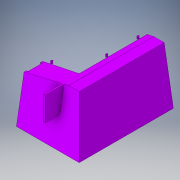
# Autodesk Inventor part: CPURightOne
Saved by Autodesk Inventor 2019 (Build 230136000, 136)
## iProperties
Created: 2019-01-04
Part Number: CPURightOne
Material: Generic
Document SubType Name: Modeling
Designer: james
Density: 1 g/cm^3
Appearance: Default(1)
Author: james
Autodesk Inventor part; units mm, degrees
ref_plane "YZ Plane" through (0, 0, 0) normal (1, 0, 0) x (0, 1, 0)
ref_plane "XZ Plane" through (0, 0, 0) normal (0, 1, 0) x (-1, 0, 0)
ref_plane "XY Plane" through (0, 0, 0) normal (0, 0, 1) x (1, 0, 0)
sketch "Sketch1" plane through (0, 0, 0) normal (0, 1, 0) x (-1, 0, 0)
  line L0 (8.325, 64.7833) -> (-61.525, 64.7833)
  line L1 (-61.525, 64.7833) -> (-61.525, -81.2667)
  line L2 (-61.525, -81.2667) -> (8.325, -81.2667)
  line L3 (8.325, -81.2667) -> (8.325, 64.7833)
  point P0 (0, 0)
  dimension "d0" = 146.05
  dimension "d1" = 69.85
  constraints: 8 end point, 2 parallel, 1 horizontal, 1 perpendicular
  measures "d0" distance of L0.end L1.end
  measures "d1" distance of L1.end L2.end
extrude "Extrusion1" add sketch "Sketch1" along normal blind 5.08
sketch "Sketch2" plane through (61.525, 0, 64.7833) normal (1, 0, 0) x (0, 0, -1)
  line L0 (0, 5.08) -> (146.05, 5.08) projected
  line L1 (0, 5.08) -> (5.08, 5.08)
  line L2 (5.08, 5.08) -> (5.08, 71.12)
  line L3 (5.08, 71.12) -> (0, 71.12)
  line L4 (0, 71.12) -> (0, 5.08)
  line L5 (0, 0) -> (146.05, 0) projected
  point P0 (64.7833, 0)
  dimension "d4" = 5.08
  dimension "d5" = 71.12
  constraints: 8 end point, 2 parallel, 1 horizontal, 1 perpendicular
  measures "d4" distance between parallel lines of L4 L2
  measures "d5" distance between parallel lines of L5 L3
extrude "Extrusion2" add sketch "Sketch2" against normal blind 69.85
sketch "Sketch3" plane through (61.525, 0, -81.2667) normal (0, 0, -1) x (-1, 0, 0)
  line L0 (0, 5.08) -> (69.85, 5.08) projected
  line L1 (0, 0) -> (69.85, 0) projected
  line L2 (0, 5.08) -> (5.08, 5.08)
  line L3 (5.08, 5.08) -> (5.08, 71.12)
  line L4 (5.08, 71.12) -> (0, 71.12)
  line L5 (0, 71.12) -> (0, 5.08)
  point P0 (61.525, 0)
  dimension "d8" = 5.08
  dimension "d9" = 71.12
  constraints: 8 end point, 2 parallel, 1 horizontal, 1 perpendicular
  measures "d8" distance between parallel lines of L5 L3
  measures "d9" distance between parallel lines of L1 L4
extrude "Extrusion3" add sketch "Sketch3" against normal blind 146.05
sketch "Sketch4" plane through (61.525, 71.12, 64.7833) normal (0, 1, 0) x (1, 0, 0)
  line L0 (-5.08, 5.08) -> (-69.85, 5.08) projected
  line L1 (-5.08, 146.05) -> (-5.08, 5.08) projected
  line L2 (-69.85, 5.08) -> (-5.08, 5.08) projected
  line L3 (-69.85, 5.08) -> (-69.85, -19.05)
  line L4 (-69.85, -19.05) -> (19.05, -19.05)
  line L5 (19.05, -19.05) -> (19.05, 146.05)
  line L6 (19.05, 146.05) -> (-5.08, 146.05)
  line L7 (-5.08, 5.08) -> (-5.08, 146.05) projected
  line L8 (-5.08, 5.08) -> (-5.08, 146.05)
  line L9 (-5.08, 5.08) -> (-69.85, 5.08)
  point P0 (-61.525, 64.7833)
  dimension "d12" = 24.13
  dimension "d13" = 24.13
  constraints: 12 end point, 3 perpendicular, 2 collinear, 1 vertical
  measures "d12" distance between parallel lines of L0 L4
  measures "d13" distance of L5.end L1.start
extrude "Extrusion4" add sketch "Sketch4" against normal blind 5.08
sketch "Sketch5" plane through (-8.325, 71.12, 59.7033) normal (0, 1, 0) x (1, 0, 0)
  line L0 (88.9, -24.13) -> (88.9, 140.97) projected
  line L1 (0, -24.13) -> (88.9, -24.13) projected
  point P0 (8.325, 59.7033)
  point P1 (12.7, -14.605)
  point P2 (79.375, 52.07)
  point P3 (79.375, 128.27)
  dimension "d16" = 9.525
  dimension "d17" = 9.525
  dimension "d18" = 76.2
  dimension "d19" = 76.2
  dimension "d20" = 9.525
  dimension "d21" = 76.2
  measures "d16" distance from line of L0 point (79.375, 52.07)
  measures "d17" distance from line of L1 point (12.7, -14.605)
  measures "d18" distance from line of point (12.7, -14.605) L0
  measures "d19" distance from line of L1 point (79.375, 52.07)
  measures "d20" distance from line of L0 point (79.375, 128.27)
  measures "d21" distance of point (79.375, 52.07) point (79.375, 128.27)
hole "Hole1" at (4.375, 71.12, 74.3083) at (71.05, 71.12, 7.6333) at (71.05, 71.12, -68.5667) direction (0, -1, 0) diameter 4.826 end through all
sketch "Sketch6" plane through (-8.325, 0, -81.2667) normal (-1, 0, 0) x (0, 0, 1)
  line L0 (223.52, 0) -> (228.6, 0)
  line L1 (0, 0) -> (0, 5.08) projected
  line L2 (146.05, 0) -> (146.05, 66.04) projected
  line L3 (223.52, 0) -> (201.1265, 127)
  line L4 (201.1265, 127) -> (206.2065, 127)
  line L5 (206.2065, 127) -> (228.6, 0)
  point P0 (81.2667, 0)
  dimension "d29" = 228.6
  dimension "d30" = 5.08
  dimension "d32" = 10
  dimension "d33" = 5.08
  dimension "d34" = 127
  constraints: 8 end point, 2 horizontal
  measures "d29" distance from line of L1 L0.end
  measures "d30" distance of L0.start L0.end
  measures "d32" angle of L2 L3
  measures "d33" distance of L3.end L4.end
  measures "d34" distance between parallel lines of L0 L4
extrude "Extrusion5" add sketch "Sketch6" against normal blind 152.4
sketch "Sketch7" plane through (61.525, 0, -81.2667) normal (0, 0, -1) x (-1, 0, 0)
  line L0 (-82.55, 0) -> (-77.47, 0)
  line L1 (69.85, 0) -> (-82.55, 0) projected
  line L2 (-77.47, 0) -> (-55.0765, 127)
  line L3 (0, 0) -> (0, 66.04) projected
  line L4 (69.85, 127) -> (-82.55, 127) projected
  line L5 (-55.0765, 127) -> (-60.1565, 127)
  line L6 (-60.1565, 127) -> (-82.55, 0)
  point P0 (61.525, 0)
  dimension "d37" = 5.08
  dimension "d38" = 10
  dimension "d39" = 5.08
  constraints: 8 end point, 3 point on line
  measures "d37" distance of L0.start L0.end
  measures "d38" angle of L2 L3
  measures "d39" distance of L5.end L2.end
extrude "Extrusion6" add sketch "Sketch7" against normal blind 228.6
sketch "Sketch8" plane through (61.525, 0, -81.2667) normal (0, 0, -1) x (-1, 0, 0)
  line L0 (-60.1565, 127) -> (-82.55, 0) projected
  line L1 (-60.1565, 127) -> (-82.55, 127) projected
  line L2 (-82.55, 0) -> (-82.55, 127) projected
  point P0 (61.525, 0)
extrude "Extrusion7" cut sketch "Sketch8" against normal blind 228.6
sketch "Sketch9" plane through (-8.325, 0, -81.2667) normal (-1, 0, 0) x (0, 0, 1)
  line L0 (228.6, 0) -> (206.2065, 127) projected
  line L1 (206.2065, 127) -> (228.6, 127) projected
  line L2 (228.6, 127) -> (228.6, 0) projected
  point P0 (81.2667, 0)
extrude "Extrusion8" cut sketch "Sketch9" against normal blind 228.6
sketch "Sketch10" plane through (61.525, 0, -81.2667) normal (0, 0, -1) x (-1, 0, 0)
  line L0 (-60.1565, 127) -> (-82.55, 0) projected
  line L1 (-60.1565, 127) -> (-34.7565, 127)
  line L2 (-34.7565, 127) -> (-34.7565, 121.92)
  line L3 (-34.7565, 121.92) -> (-60.1565, 121.92)
  line L4 (-60.1565, 121.92) -> (-60.1565, 127)
  point P0 (61.525, 0)
  dimension "d46" = 25.4
  dimension "d47" = 5.08
  constraints: 8 end point, 2 parallel, 1 horizontal, 1 perpendicular
  measures "d46" distance of L2.end L3.end
  measures "d47" distance between parallel lines of L3 L1
extrude "Extrusion9" add sketch "Sketch10" against normal blind 204.7875
sketch "Sketch13" plane through (61.525, 0, -81.2667) normal (0, 0, -1) x (-1, 0, 0)
  line L0 (-34.7565, 127) -> (-60.1565, 127) projected
  line L1 (-34.7565, 127) -> (65.3895, 106.1149)
  line L2 (65.3895, 106.1149) -> (65.3895, 101.0349)
  line L3 (-34.7565, 127) -> (-34.7565, 121.92) projected
  line L4 (-34.7565, 127) -> (-34.7565, 121.92)
  line L5 (-34.7565, 121.92) -> (65.3895, 101.0349)
  point P0 (61.525, 0)
  dimension "d50" = 5.08
  dimension "d51" = 168.22
  constraints: 8 end point, 1 collinear, 1 perpendicular
  measures "d50" distance of L1.end L2.end
  measures "d51" angle of L0 L1
extrude "Extrusion10" add sketch "Sketch13" against normal blind 204.7875
sketch "Sketch14" plane through (-8.325, 0, -81.2667) normal (-1, 0, 0) x (0, 0, 1)
  line L0 (0, 66.04) -> (165.1, 66.04) projected
  line L1 (165.1, 66.04) -> (170.18, 66.04)
  line L2 (170.18, 66.04) -> (170.18, 144.8486)
  line L3 (165.1, 66.04) -> (165.1, 144.8486)
  line L4 (165.1, 144.8486) -> (170.18, 144.8486)
  point P0 (81.2667, 0)
  dimension "d54" = 5.08
  constraints: 8 end point, 2 perpendicular, 1 horizontal, 1 vertical
  measures "d54" distance between parallel lines of L2 L3
extrude "Extrusion11" add sketch "Sketch14" against normal blind 201.6125
sketch "Sketch15" plane through (61.525, 0, -81.2667) normal (0, 0, -1) x (-1, 0, 0)
  line L0 (-19.05, 66.04) -> (-65.8254, 66.04) projected
  line L1 (-19.05, 66.04) -> (-24.13, 66.04)
  line L2 (-24.13, 66.04) -> (-24.13, 144.9245)
  line L3 (-24.13, 144.9245) -> (-19.05, 144.9245)
  line L4 (-19.05, 144.9245) -> (-19.05, 66.04)
  point P0 (61.525, 0)
  dimension "d57" = 5.08
  constraints: 8 end point, 2 parallel, 1 horizontal, 1 perpendicular
  measures "d57" distance between parallel lines of L2 L4
extrude "Extrusion12" add sketch "Sketch15" against normal blind 252.4125
sketch "Sketch18" plane through (-8.325, 71.12, 83.8333) normal (0, 0, -1) x (-1, 0, 0)
  line L0 (-4.4605, 34.9949) -> (-88.9, 52.6045) projected
  line L1 (-88.9, 52.6045) -> (26.3817, 28.5629)
  line L2 (-88.9, 52.6045) -> (-88.9, 80.9754)
  line L3 (-88.9, 80.9754) -> (26.3817, 80.9754)
  line L4 (26.3817, 80.9754) -> (26.3817, 28.5629)
  point P0 (-8.325, -71.12)
  constraints: 8 end point, 2 perpendicular, 1 collinear, 1 vertical
extrude "Extrusion14" cut sketch "Sketch18" against normal blind 133.35
sketch "Sketch19" plane through (61.525, 0, -81.2667) normal (0, 0, -1) x (-1, 0, 0)
  line L0 (-19.05, 66.04) -> (-19.05, 123.7245) projected
  line L1 (-24.13, 124.7839) -> (-34.7565, 127) projected
  line L2 (-19.05, 123.7245) -> (-34.7565, 127)
  line L3 (-34.7565, 127) -> (-82.8145, 127)
  line L4 (-82.8145, 127) -> (-82.8145, 152.1406)
  line L5 (-82.8145, 152.1406) -> (-18.2912, 151.7847)
  line L6 (-18.2912, 151.7847) -> (-19.05, 123.7245)
  point P0 (61.525, 0)
  constraints: 10 end point, 1 collinear, 1 horizontal, 1 perpendicular
extrude "Extrusion15" cut sketch "Sketch19" against normal blind 338.1375
sketch "Sketch21" plane through (0, 5.08, 0) normal (0, 1, 0) x (1, 0, 0)
  line L0 (56.445, -59.7033) -> (56.445, 81.2667) projected
  line L1 (56.445, 81.2667) -> (-8.325, 81.2667) projected
  line L2 (-8.325, 81.2667) -> (-8.325, -59.7033) projected
  line L3 (-8.325, -59.7033) -> (56.445, -59.7033) projected
  point P0 (0, 0)
extrude "Extrusion16" cut sketch "Sketch21" along normal blind 338.1375
sketch "Sketch22" plane through (-8.325, 71.12, 59.7033) normal (0, 1, 0) x (1, 0, 0)
  circle A0 centre (79.375, 52.07) radius 2.413 projected
  circle A1 centre (12.7, -14.605) radius 2.413 projected
  circle A2 centre (79.375, 128.27) radius 2.413 projected
  line L0 (64.77, 0) -> (0, 0) projected
  line L1 (0, 0) -> (0, -24.13) projected
  line L2 (0, -24.13) -> (88.9, -24.13) projected
  line L3 (88.9, -24.13) -> (88.9, 140.97) projected
  line L4 (64.77, 140.97) -> (88.9, 140.97) projected
  line L5 (64.77, 140.97) -> (64.77, 0) projected
  point P0 (8.325, 59.7033)
extrude "Extrusion17" cut sketch "Sketch22" along normal blind 338.1375
sketch "Sketch23" plane through (193.2875, 66.04, 83.8333) normal (0, 0, -1) x (-1, 0, 0)
  line L0 (60.8571, 0) -> (0, 0) projected
  line L1 (60.8571, 0) -> (76.6392, 89.5043)
  line L2 (71.606, 60.96) -> (49.2125, -66.04) projected
  line L3 (76.6392, 89.5043) -> (-29.2639, 89.5043)
  line L4 (-29.2639, 89.5043) -> (-29.2639, 0)
  line L5 (-29.2639, 0) -> (60.8571, 0)
  point P0 (193.2875, -66.04)
  constraints: 8 end point, 2 perpendicular, 1 collinear, 1 horizontal
extrude "Extrusion18" cut sketch "Sketch23" against normal blind 338.1375
equation "\"d0\" = DU1CHLength"
equation "\"d1\" = DU1CHWidth"
equation "\"d2\" = WallWidth"
equation "\"d4\" = WallWidth"
equation "\"d5\" = CPDeckHeight"
equation "\"d6\" = DU1CHWidth"
equation "\"d8\" = WallWidth"
equation "\"d9\" = CPDeckHeight"
equation "\"d10\" = DU1CHLength"
equation "\"d12\" = WallWidth + ControlPlateShelfLength"
equation "\"d13\" = WallWidth + ControlPlateShelfLength"
equation "\"d14\" = WallWidth"
equation "\"d16\" = ControlHoleBoltHoleMid"
equation "\"d17\" = ControlHoleBoltHoleMid"
equation "\"d18\" = ControlPlateScrewLength"
equation "\"d19\" = ControlPlateScrewLength"
equation "\"d20\" = ControlHoleBoltHoleMid"
equation "\"d21\" = ControlPlateScrewLength"
equation "\"d29\" = PartLength"
equation "\"d30\" = WallWidth"
equation "\"d32\" = EdgeAngle"
equation "\"d33\" = WallWidth"
equation "\"d34\" = DSBackHeight"
equation "\"d35\" = PartWidth"
equation "\"d37\" = WallWidth"
equation "\"d38\" = EdgeAngle"
equation "\"d39\" = WallWidth"
equation "\"d40\" = PartLength"
equation "\"d42\" = PartLength"
equation "\"d44\" = PartLength"
equation "\"d46\" = BackShelf"
equation "\"d47\" = WallWidth"
equation "\"d50\" = WallWidth"
equation "\"d51\" = MainAngle"
equation "\"d54\" = WallWidth"
equation "\"d57\" = WallWidth"
equation "\"DSLength\" = 1371.6"
equation "\"DSWidth\" = 304.8"
equation "\"DCDeckHeight\" = 76.2"
equation "\"WallWidth\" = 5.08"
equation "\"EdgeAngle\" = 10deg"
equation "\"LengthCuts\" = 152.4"
equation "\"WidthCuts\" = 50.8"
equation "\"PartLength\" = 228.6"
equation "\"PartWidth\" = 152.4"
equation "\"BoltHoldDiam\" = 6.35"
equation "\"ControlPlateLength\" = 228.6"
equation "\"ControlPlateWidth\" = 228.6"
equation "\"ControlPlateShelfLength\" = 19.05"
equation "\"ControlHoleLength\" = 190.5"
equation "\"ControlHoleWidth\" = 190.5"
equation "\"ControlHoleFromSide\" = 63.5"
equation "\"ControlHoleBoltHoleMid\" = 9.525"
equation "\"DU1CHWidth\" = 69.85"
equation "\"CPFromSide\" = 63.5"
equation "\"CPFromBack\" = 63.5"
equation "\"DU1CHLength\" = 146.05"
equation "\"CPDeckHeight\" = 71.12"
equation "\"ControlPlateScrewLength\" = 76.2"
equation "\"DSBackHeight\" = 127"
equation "\"BackShelf\" = 25.4"
equation "\"MainAngle\" = 168.22deg"
equation "\"CPDWidthHole\" = 120.65"
equation "\"CPDLengthHole\" = 146.05"
equation "\"DownBackHeight\" = 130.7084"
body "Solid1"
